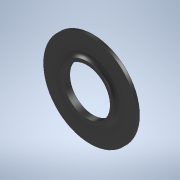
# Autodesk Inventor part: Retenedor
Saved by Autodesk Inventor 2022 (Build 260153000, 153)
## iProperties
Created: 2021-02-18
Part Number: Retenedor
Material: Generic
Document SubType Name: Modeling
Designer: juanp
Density: 1 g/cm^3
Appearance: Glossy - Black
Author: juanp
Autodesk Inventor part; units mm, degrees
ref_plane "YZ Plane" through (0, 0, 0) normal (1, 0, 0) x (0, 1, 0)
ref_plane "XZ Plane" through (0, 0, 0) normal (0, 1, 0) x (-1, 0, 0)
ref_plane "XY Plane" through (0, 0, 0) normal (0, 0, 1) x (1, 0, 0)
sketch "Sketch1" plane through (0, 0, 0) normal (0, 0, 1) x (1, 0, 0)
  circle A0 centre (0, 0) radius 7.5
  circle A1 centre (0, 0) radius 15
  circle A2 centre (0, 0) radius 8.5
  dimension "d0" = 15
  dimension "d1" = 30
  dimension "d2" = 1
  constraints: 3 centre point, 3 coincident
  measures "d0" diameter of A0
  measures "d1" diameter of A1
  measures "d2" radial gap between concentric circles of A2 A0
extrude "Extrusion1" add sketch "Sketch1" along normal blind 1 contours A1
extrude "Extrusion2" add sketch "Sketch1" along normal blind 2 contours A2
fillet "Fillet1" radius 2 1 edges at (-8.5, 0, 1)
body "Solid1"
